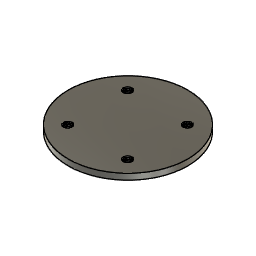
rod_blockoff (Autodesk Fusion 360 design; units mm, degrees)
Autodesk Fusion 360 part; units mm, degrees
sketch "Sketch1" plane through (0, 0, 0) normal (0, 0, 1) x (1, 0, 0)
  circle A0 centre (0, 0) radius 20
  dimension "d1" = 40
  constraint coincident A0.centre origin
  measures "d1" diameter of A0
extrude "Extrude1" add sketch "Sketch1" along normal blind 2
sketch "Sketch2" plane through (0, 0, 2) normal (0, 0, 1) x (-1, 0, 0)
  circle A0 centre (0, 0) radius 20
  line L0 (10, -10) -> (-10, -10) construction
  line L1 (-10, -10) -> (-10, 10) construction
  line L2 (-10, 10) -> (10, 10) construction
  line L3 (10, 10) -> (10, -10) construction
  circle A1 centre (10, -10) radius 1.5
  circle A2 centre (-10, -10) radius 1.5
  circle A3 centre (10, 10) radius 1.5
  circle A4 centre (-10, 10) radius 1.5
  dimension "d4" = 10
  dimension "d5" = 10
  dimension "d6" = 3
  dimension "d7" = 3
  dimension "d8" = 3
  dimension "d9" = 3
  constraint horizontal L0
  constraint vertical L1
  constraint horizontal L2
  constraint vertical L3
  constraint coincident L0.start L3.end
  constraint coincident L0.end L1.start
  constraint coincident L2.end L3.start
  constraint coincident L1.end L2.start
  measures "d4" distance of A0.centre L2
  measures "d5" distance of A0.centre L1
  measures "d6" diameter of A1
  measures "d7" diameter of A2
  measures "d8" diameter of A3
  measures "d9" diameter of A4
hole "Hole1" at (-10, -10, 2) at (-10, 10, 2) at (10, 10, 2) at (10, -10, 2) direction (0, 0, -1) diameter 2.529 depth 2 tip angle 118
thread "Thread1" "ISO Metric profile 3.0 M3x0.5 M3x0.5 6H" major diameter 3.086 minor diameter 2.529 pitch 0.5 angle 60 modelled right hand crest width 0.1368 on face at (-9.8741, 8.7418, 1.3333) crest through (-8.7355, 10, 1.875) on face at (10.1259, -11.2582, 1.3333) crest through (11.2645, -10, 1.875) on face at (10.1259, 8.7418, 1.3333) crest through (11.2645, 10, 1.875) on face at (-9.8741, -11.2582, 1.3333) crest through (-8.7355, -10, 1.875)
